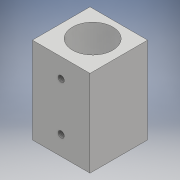
# Autodesk Inventor part: blocoSuporteRolamentosTeste
Saved by Autodesk Inventor 2018 (Build 220112000, 112)
## iProperties
Created: 2018-08-27
Part Number: blocoSuporteRolamentosTeste
Material: Genérico
Document SubType Name: Modeling
Designer: Georgines
Density: 1 g/cm^3
Appearance: Padrão
Author: Georgines
Autodesk Inventor part; units mm, degrees
ref_plane "YZ Plane" through (0, 0, 0) normal (1, 0, 0) x (0, 1, 0)
ref_plane "XZ Plane" through (0, 0, 0) normal (0, 1, 0) x (-1, 0, 0)
ref_plane "XY Plane" through (0, 0, 0) normal (0, 0, 1) x (1, 0, 0)
sketch "Esboço2" plane through (0, 0, 0) normal (0, 0, 1) x (1, 0, 0)
  line L0 (-15, 10) -> (15, 10)
  line L1 (15, 10) -> (15, -20)
  line L2 (15, -20) -> (-15, -20)
  line L3 (-15, -20) -> (-15, 10)
  line L4 (-15, 10) -> (15, -20) construction
  line L5 (15, 10) -> (-15, -20) construction
  point P0 (0, -5)
  dimension "d10" = 30
  dimension "d11" = 30
  constraints: 12 end point, 2 midpoint, 2 parallel, 1 horizontal, 1 perpendicular
  measures "d10" distance of L1.end L2.end
  measures "d11" distance of L0.end L1.end
extrude "Extrusão1" add sketch "Esboço2" along normal blind 45
sketch "Esboço3" plane through (0, 0, 45) normal (0, 0, 1) x (1, 0, 0)
  line L0 (15, 10) -> (-15, 10) projected
  line L1 (0, 10) -> (0, -3.62)
  circle A0 centre (0, -3.62) radius 10.5
  point P0 (0, 0)
  dimension "d14" = 13.62
  dimension "d15" = 21
  constraints: 2 end point, 1 centre point, 1 coincident, 1 midpoint, 1 vertical
  measures "d14" distance of L1.start L1.end
  measures "d15" diameter of A0
hole "Furo1" at (0, -3.62, 45) direction (0, 0, -1) diameter 12.5 end through all counterbore diameter 21 counterbore depth 32
sketch "Esboço4" plane through (-15, -20, 0) normal (0, -1, 0) x (1, 0, 0)
  line L0 (15, 0) -> (15, 45)
  line L1 (30, 45) -> (0, 45) projected
  circle A0 centre (15, 10) radius 1.6056 construction
  circle A1 centre (15, 35) radius 1.4692 construction
  line L2 (0, 0) -> (0, 45) construction
  line L3 (0, 22.5) -> (30, 22.5) construction
  line L4 (30, 0) -> (30, 45) construction
  dimension "d23" = 12.5
  dimension "d24" = 12.5
  constraints: 4 end point, 3 midpoint, 2 centre point, 2 point on line
  measures "d23" distance from line of A0.centre L3
  measures "d24" distance from line of A1.centre L3
hole "Furo2" at (0, -20, 10) at (0, -20, 35) direction (0, 1, 0) diameter 3.242 depth 6 tip angle 118 thread size "M4x0.7" class "6H" standard "ANSI Metric M Profile"
